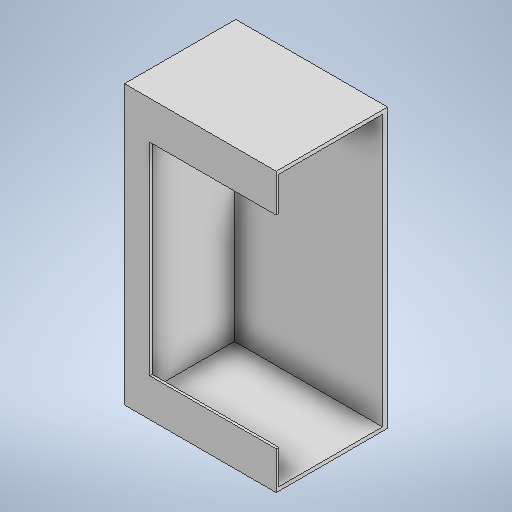
# Autodesk Inventor part: Intake_I2D_Bottom
Saved by Autodesk Inventor 2025 (Build 290162010, 162A)
## iProperties
Created: 2024-10-13
Part Number: Intake_I2D_Bottom
Material: Generic
Document SubType Name: Modeling
Designer: dcfam
Density: 1 g/cm^3
Appearance: Default
Author: dcfam
Autodesk Inventor part; units mm, degrees
ref_plane "YZ Plane" through (0, 0, 0) normal (1, 0, 0) x (0, 1, 0)
ref_plane "XZ Plane" through (0, 0, 0) normal (0, 1, 0) x (-1, 0, 0)
ref_plane "XY Plane" through (0, 0, 0) normal (0, 0, 1) x (1, 0, 0)
sketch "Sketch1" plane through (0, 0, 0) normal (0, 0, 1) x (1, 0, 0)
  line L0 (-30, -55) -> (30, -55)
  line L1 (30, -55) -> (30, 55)
  line L2 (30, 55) -> (-30, 55)
  line L3 (-30, 55) -> (-30, -55)
  line L4 (-30, -55) -> (30, 55) construction
  line L5 (30, -55) -> (-30, 55) construction
  point P0 (0, 0)
  dimension "d0" = 60
  dimension "d1" = 110
  constraints: 12 end point, 2 midpoint, 2 parallel, 1 horizontal, 1 perpendicular
  measures "d0" distance of L2.end L1.end
  measures "d1" distance of L1.end L0.end
extrude "Extrusion1" add sketch "Sketch1" along normal blind 2
sketch "Sketch2" plane through (0, 0, 2) normal (0, 0, 1) x (1, 0, 0)
  line L0 (30, -55) -> (30, 55) projected
  line L1 (30, 55) -> (-30, 55) projected
  line L2 (-30, 55) -> (-30, -55) projected
  line L3 (-30, -55) -> (30, -55) projected
  line L4 (28.5, 53.5) -> (-28.5, 53.5)
  line L5 (-28.5, 53.5) -> (-28.5, -53.5)
  line L6 (-28.5, -53.5) -> (28.5, -53.5)
  line L7 (28.5, -53.5) -> (30, -53.5)
  line L8 (30, -55) -> (30, 55) projected
  line L9 (30, -53.5) -> (30, -55)
  line L10 (28.5, 53.5) -> (30, 53.5)
  line L11 (30, 53.5) -> (30, 55)
  line L12 (30, 55) -> (-30, 55)
  line L13 (-30, 55) -> (-30, -55)
  line L14 (-30, -55) -> (30, -55)
  point P0 (0, 0)
  dimension "d4" = 1.5
  constraints: 20 end point, 4 perpendicular, 2 collinear, 2 point on line, 1 horizontal, 2 other
  measures "d4" distance between parallel lines of L3 L6
extrude "Extrusion2" add sketch "Sketch2" along normal blind 42 contours L3 L2 L1 L0 L10 L4 L5 L6 L7
sketch "Sketch3" plane through (0, 0, 44) normal (0, 0, 1) x (1, 0, 0)
  line L0 (-30, -55) -> (30, -55) projected
  line L1 (30, 55) -> (-30, 55) projected
  line L2 (-30, -55) -> (30, -55)
  line L3 (30, -55) -> (30, 55)
  line L4 (30, 55) -> (-30, 55)
  line L5 (-30, 55) -> (-30, -55)
  point P0 (0, 0)
  constraints: 8 end point, 2 parallel, 1 horizontal, 1 perpendicular
extrude "Extrusion3" add sketch "Sketch3" against normal blind 1
sketch "Sketch4" plane through (0, 0, 44) normal (0, 0, 1) x (1, 0, 0)
  line L0 (20, -40) -> (-20, -40)
  line L1 (-20, -40) -> (-20, 40)
  line L2 (-20, 40) -> (20, 40)
  line L3 (20, -40) -> (-20, 40) construction
  line L4 (-20, -40) -> (20, 40) construction
  line L5 (20, -40) -> (30, -40)
  line L6 (30, 53.5) -> (30, -53.5) projected
  line L7 (20, 40) -> (30, 40)
  line L8 (30, 40) -> (30, -40)
  line L9 (30, -40) -> (30, 40)
  point P0 (0, 0)
  dimension "d9" = 40
  dimension "d10" = 80
  constraints: 18 end point, 3 horizontal, 2 midpoint, 2 perpendicular, 1 collinear, 1 parallel, 1 point on line
  measures "d9" distance of L1.end L2.end
  measures "d10" distance of L0.end L1.end
extrude "Extrusion4" cut sketch "Sketch4" against normal blind 10.525
body "Solid1"
